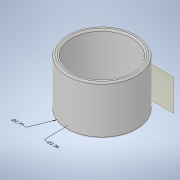
# Autodesk Inventor part: LargeFinderObjectiveCover-V02
Saved by Autodesk Inventor 2021.1 (Build 251245010, 245A)
## iProperties
Created: 2018-09-01
Part Number: LargeFinderObjectiveCover-V02
Material: Generic
Document SubType Name: Modeling
Designer: steele
Density: 1 g/cm^3
Appearance: Default
Author: steele
Autodesk Inventor part; units mm, degrees
ref_plane "YZ Plane" through (0, 0, 0) normal (1, 0, 0) x (0, 1, 0)
ref_plane "XZ Plane" through (0, 0, 0) normal (0, 1, 0) x (-1, 0, 0)
sketch "Sketch1" plane through (0, 0, 0) normal (0, 1, 0) x (-1, 0, 0)
  circle A0 centre (0, 0) radius 35.1155
  dimension "d0" = 70.231
  constraints: 1 centre point, 1 coincident
  measures "d0" diameter of A0
extrude "Extrusion1" add sketch "Sketch1" along normal blind 4.7625
sketch "Sketch2" plane through (0, 4.7625, 0) normal (0, 1, 0) x (1, 0, 0)
  circle A0 centre (0, 0) radius 35.1155
  circle A1 centre (0, 0) radius 30.353
  dimension "d4" = 60.706
  dimension "d5" = 70.231
  constraints: 2 centre point, 1 coincident
  measures "d4" diameter of A1
  measures "d5" diameter of A0
extrude "Extrusion3" add sketch "Sketch2" along normal blind 44.45
ref_plane "Work Plane1" through (0, 0, -35.1155) normal (0, 0, 1) x (1, 0, 0)
sketch "Sketch5" plane through (0, 0, -35.1155) normal (0, 0, 1) x (1, 0, 0)
  line L0 (-35.1155, 0) -> (-35.1155, 49.2125) projected
  line L1 (35.1155, 0) -> (35.1155, 49.2125) projected
  line L2 (35.1155, 24.6063) -> (-35.1155, 24.6063) construction
  line L3 (-14.5772, 19.5263) -> (-16.545, 19.5263)
  line L4 (-16.545, 19.5263) -> (-16.545, 19.0075)
  line L5 (-16.545, 19.0075) -> (-15.8987, 19.0075)
  line L6 (-15.8987, 19.0075) -> (-15.8987, 14.965)
  line L7 (-15.8987, 14.965) -> (-16.545, 14.965)
  line L8 (-16.545, 14.965) -> (-16.545, 14.4462)
  line L9 (-16.545, 14.4462) -> (-14.5772, 14.4462)
  line L10 (-14.5772, 14.4462) -> (-14.5772, 14.965)
  line L11 (-14.5772, 14.965) -> (-15.2235, 14.965)
  line L12 (-15.2235, 14.965) -> (-15.2235, 19.0075)
  line L13 (-15.2235, 19.0075) -> (-14.5772, 19.0075)
  line L14 (-14.5772, 19.0075) -> (-14.5772, 19.5263)
  spline S0 degree 2 poles (-9.736, 16.9904) (-9.736, 17.6861) (-10.3, 18.8058) (-10.7734, 19.1187) knots 0 0 0 1 2 2 2
  spline S1 degree 2 poles (-10.7734, 19.1187) (-11.1604, 19.3616) (-11.9549, 19.5263) (-12.5724, 19.5263) knots 0 0 0 1 2 2 2
  line L15 (-12.5724, 19.5263) -> (-13.7415, 19.5263)
  line L16 (-13.7415, 19.5263) -> (-13.7415, 14.4462)
  line L17 (-13.7415, 14.4462) -> (-12.5847, 14.4462)
  spline S2 degree 2 poles (-12.5847, 14.4462) (-11.8684, 14.4462) (-11.0533, 14.6603) (-10.7652, 14.8497) knots 0 0 0 1 2 2 2
  spline S3 degree 2 poles (-10.7652, 14.8497) (-10.2753, 15.1749) (-9.736, 16.2494) (-9.736, 16.9904) knots 0 0 0 1 2 2 2
  spline S4 degree 2 poles (-10.4399, 16.9821) (-10.4399, 16.3976) (-10.8269, 15.5701) (-11.2098, 15.3355) knots 0 0 0 1 2 2 2
  spline S5 degree 2 poles (-11.2098, 15.3355) (-11.4815, 15.1749) (-12.0948, 15.0308) (-12.5518, 15.0308) knots 0 0 0 1 2 2 2
  line L18 (-12.5518, 15.0308) -> (-13.0664, 15.0308)
  line L19 (-13.0664, 15.0308) -> (-13.0664, 18.9417)
  line L20 (-13.0664, 18.9417) -> (-12.5518, 18.9417)
  spline S6 degree 2 poles (-12.5518, 18.9417) (-12.1031, 18.9417) (-11.4238, 18.7976) (-11.148, 18.6041) knots 0 0 0 1 2 2 2
  spline S7 degree 2 poles (-11.148, 18.6041) (-10.794, 18.3653) (-10.4399, 17.5749) (-10.4399, 16.9821) knots 0 0 0 1 2 2 2
  line L21 (-3.5115, 19.5263) -> (-4.3266, 19.5263)
  line L22 (-4.3266, 19.5263) -> (-4.3266, 18.5547)
  line L23 (-4.3266, 18.5547) -> (-3.5115, 18.5547)
  line L24 (-3.5115, 18.5547) -> (-3.5115, 19.5263)
  line L25 (-3.5115, 16.6857) -> (-4.3266, 16.6857)
  line L26 (-4.3266, 16.6857) -> (-4.3266, 15.7142)
  line L27 (-4.3266, 15.7142) -> (-3.5115, 15.7142)
  line L28 (-3.5115, 15.7142) -> (-3.5115, 16.6857)
  line L29 (3.0011, 19.5263) -> (-0.1317, 19.5263)
  line L30 (-0.1317, 19.5263) -> (-0.1317, 18.8058)
  spline S8 degree 2 poles (-0.1317, 18.8058) (0.2058, 18.4888) (0.8069, 17.9002) (1.095, 17.5832) knots 0 0 0 1 2 2 2
  spline S9 degree 2 poles (1.095, 17.5832) (1.6755, 16.9451) (2.0995, 16.1794) (2.0995, 15.7718) knots 0 0 0 1 2 2 2
  spline S10 degree 2 poles (2.0995, 15.7718) (2.0995, 15.5578) (1.9678, 15.2367) (1.8484, 15.1337) knots 0 0 0 1 2 2 2
  spline S11 degree 2 poles (1.8484, 15.1337) (1.729, 15.0308) (1.4161, 14.9279) (1.2268, 14.9279) knots 0 0 0 1 2 2 2
  spline S12 degree 2 poles (1.2268, 14.9279) (1.0456, 14.9279) (0.6751, 15.0185) (0.5064, 15.0885) knots 0 0 0 1 2 2 2
  spline S13 degree 2 poles (0.5064, 15.0885) (0.3623, 15.1461) (0.0947, 15.3108) (0.0123, 15.3684) knots 0 0 0 1 2 2 2
  line L31 (0.0123, 15.3684) -> (-0.0247, 15.3684)
  line L32 (-0.0247, 15.3684) -> (-0.0247, 14.6439)
  spline S14 degree 2 poles (-0.0247, 14.6439) (0.1853, 14.5409) (0.9386, 14.3392) (1.2762, 14.3392) knots 0 0 0 1 2 2 2
  spline S15 degree 2 poles (1.2762, 14.3392) (1.9884, 14.3392) (2.7911, 15.0926) (2.7911, 15.7348) knots 0 0 0 1 2 2 2
  spline S16 degree 2 poles (2.7911, 15.7348) (2.7911, 16.0353) (2.6512, 16.5375) (2.5276, 16.7516) knots 0 0 0 1 2 2 2
  spline S17 degree 2 poles (2.5276, 16.7516) (2.4041, 16.9739) (2.046, 17.4103) (1.8484, 17.6202) knots 0 0 0 1 2 2 2
  spline S18 degree 2 poles (1.8484, 17.6202) (1.5273, 17.9701) (0.741, 18.7194) (0.5064, 18.9376) knots 0 0 0 1 2 2 2
  line L33 (0.5064, 18.9376) -> (3.0011, 18.9376)
  line L34 (3.0011, 18.9376) -> (3.0011, 19.5263)
  line L35 (4.7712, 19.5263) -> (3.9561, 19.5263)
  line L36 (3.9561, 19.5263) -> (3.9561, 18.5547)
  line L37 (3.9561, 18.5547) -> (4.7712, 18.5547)
  line L38 (4.7712, 18.5547) -> (4.7712, 19.5263)
  spline S19 degree 2 poles (7.1672, 14.9279) (6.9819, 14.9279) (6.6155, 15.0185) (6.4385, 15.0885) knots 0 0 0 1 2 2 2
  spline S20 degree 2 poles (6.4385, 15.0885) (6.2738, 15.1584) (6.031, 15.3066) (5.9363, 15.3725) knots 0 0 0 1 2 2 2
  line L39 (5.9363, 15.3725) -> (5.8951, 15.3725)
  line L40 (5.8951, 15.3725) -> (5.8951, 14.6521)
  spline S21 degree 2 poles (5.8951, 14.6521) (6.1174, 14.5327) (6.879, 14.3392) (7.2207, 14.3392) knots 0 0 0 1 2 2 2
  spline S22 degree 2 poles (7.2207, 14.3392) (7.5665, 14.3392) (8.0811, 14.4792) (8.291, 14.6274) knots 0 0 0 1 2 2 2
  spline S23 degree 2 poles (8.291, 14.6274) (8.5133, 14.7879) (8.7439, 15.2531) (8.7439, 15.566) knots 0 0 0 1 2 2 2
  spline S24 degree 2 poles (8.7439, 15.566) (8.7439, 15.9859) (8.1922, 16.6199) (7.8053, 16.7022) knots 0 0 0 1 2 2 2
  line L41 (7.8053, 16.7022) -> (7.8053, 16.7516)
  spline S25 degree 2 poles (7.8053, 16.7516) (7.9658, 16.7845) (8.3322, 16.9327) (8.4886, 17.0809) knots 0 0 0 1 2 2 2
  spline S26 degree 2 poles (8.4886, 17.0809) (8.6451, 17.225) (8.8427, 17.6861) (8.8427, 18.0195) knots 0 0 0 1 2 2 2
  spline S27 degree 2 poles (8.8427, 18.0195) (8.8427, 18.3612) (8.608, 18.9417) (8.3939, 19.164) knots 0 0 0 1 2 2 2
  spline S28 degree 2 poles (8.3939, 19.164) (8.1716, 19.3945) (7.5418, 19.6333) (7.1425, 19.6333) knots 0 0 0 1 2 2 2
  spline S29 degree 2 poles (7.1425, 19.6333) (6.7596, 19.6333) (6.0104, 19.448) (5.7551, 19.3204) knots 0 0 0 1 2 2 2
  line L42 (5.7551, 19.3204) -> (5.7551, 18.6)
  line L43 (5.7551, 18.6) -> (5.8045, 18.6)
  spline S30 degree 2 poles (5.8045, 18.6) (6.0186, 18.7564) (6.7431, 19.0446) (7.1013, 19.0446) knots 0 0 0 1 2 2 2
  spline S31 degree 2 poles (7.1013, 19.0446) (7.3112, 19.0446) (7.7312, 18.9129) (7.8711, 18.7605) knots 0 0 0 1 2 2 2
  spline S32 degree 2 poles (7.8711, 18.7605) (8.007, 18.6082) (8.1511, 18.246) (8.1511, 17.9701) knots 0 0 0 1 2 2 2
  spline S33 degree 2 poles (8.1511, 17.9701) (8.1511, 17.6943) (7.9905, 17.3362) (7.8464, 17.2333) knots 0 0 0 1 2 2 2
  spline S34 degree 2 poles (7.8464, 17.2333) (7.7023, 17.1303) (7.3112, 17.0521) (7.0807, 17.0521) knots 0 0 0 1 2 2 2
  line L44 (7.0807, 17.0521) -> (6.7925, 17.0521)
  line L45 (6.7925, 17.0521) -> (6.7925, 16.4881)
  line L46 (6.7925, 16.4881) -> (7.019, 16.4881)
  spline S35 degree 2 poles (7.019, 16.4881) (7.4759, 16.4881) (8.0523, 16.0518) (8.0523, 15.636) knots 0 0 0 1 2 2 2
  spline S36 degree 2 poles (8.0523, 15.636) (8.0523, 15.4425) (7.9041, 15.1667) (7.7847, 15.0843) knots 0 0 0 1 2 2 2
  spline S37 degree 2 poles (7.7847, 15.0843) (7.6571, 14.9979) (7.3442, 14.9279) (7.1672, 14.9279) knots 0 0 0 1 2 2 2
  spline S38 degree 2 poles (9.4684, 16.097) (9.4684, 15.706) (9.7236, 15.0555) (9.9459, 14.8209) knots 0 0 0 1 2 2 2
  spline S39 degree 2 poles (9.9459, 14.8209) (10.1559, 14.5945) (10.7693, 14.3433) (11.0821, 14.3433) knots 0 0 0 1 2 2 2
  spline S40 degree 2 poles (11.0821, 14.3433) (11.4321, 14.3433) (12.0002, 14.578) (12.2101, 14.8003) knots 0 0 0 1 2 2 2
  spline S41 degree 2 poles (12.2101, 14.8003) (12.4736, 15.0802) (12.7618, 15.9859) (12.7618, 16.6816) knots 0 0 0 1 2 2 2
  spline S42 degree 2 poles (12.7618, 16.6816) (12.7618, 17.3115) (12.4777, 18.4394) (12.2019, 18.8141) knots 0 0 0 1 2 2 2
  spline S43 degree 2 poles (12.2019, 18.8141) (11.9096, 19.2093) (11.0863, 19.6251) (10.4852, 19.6251) knots 0 0 0 1 2 2 2
  spline S44 degree 2 poles (10.4852, 19.6251) (10.3494, 19.6251) (10.0406, 19.5962) (9.9089, 19.5551) knots 0 0 0 1 2 2 2
  line L47 (9.9089, 19.5551) -> (9.9089, 18.9005)
  line L48 (9.9089, 18.9005) -> (9.9418, 18.9005)
  spline S45 degree 2 poles (9.9418, 18.9005) (10.0283, 18.9499) (10.3905, 19.0364) (10.5758, 19.0364) knots 0 0 0 1 2 2 2
  spline S46 degree 2 poles (10.5758, 19.0364) (11.2427, 19.0364) (12.0043, 18.1554) (12.0578, 17.3403) knots 0 0 0 1 2 2 2
  spline S47 degree 2 poles (12.0578, 17.3403) (11.7861, 17.5255) (11.2921, 17.6943) (10.9998, 17.6943) knots 0 0 0 1 2 2 2
  spline S48 degree 2 poles (10.9998, 17.6943) (10.7199, 17.6943) (10.2547, 17.5708) (10.02, 17.3938) knots 0 0 0 1 2 2 2
  spline S49 degree 2 poles (10.02, 17.3938) (9.7483, 17.1839) (9.4684, 16.5458) (9.4684, 16.097) knots 0 0 0 1 2 2 2
  spline S50 degree 2 poles (12.0743, 16.5293) (12.0743, 16.0147) (11.8849, 15.3643) (11.7161, 15.1873) knots 0 0 0 1 2 2 2
  spline S51 degree 2 poles (11.7161, 15.1873) (11.5679, 15.0226) (11.2592, 14.8991) (11.078, 14.8991) knots 0 0 0 1 2 2 2
  spline S52 degree 2 poles (11.078, 14.8991) (10.6581, 14.8991) (10.16, 15.5001) (10.16, 16.0682) knots 0 0 0 1 2 2 2
  spline S53 degree 2 poles (10.16, 16.0682) (10.16, 16.3893) (10.3247, 16.8051) (10.5058, 16.9533) knots 0 0 0 1 2 2 2
  spline S54 degree 2 poles (10.5058, 16.9533) (10.6375, 17.0604) (10.9628, 17.1303) (11.1521, 17.1303) knots 0 0 0 1 2 2 2
  spline S55 degree 2 poles (11.1521, 17.1303) (11.3703, 17.1303) (11.8725, 16.978) (12.0619, 16.8504) knots 0 0 0 1 2 2 2
  spline S56 degree 2 poles (12.0619, 16.8504) (12.066, 16.801) (12.0743, 16.6322) (12.0743, 16.5293) knots 0 0 0 1 2 2 2
  spline S57 degree 2 poles (16.582, 16.9862) (16.582, 18.353) (15.7875, 19.6333) (14.9601, 19.6333) knots 0 0 0 1 2 2 2
  spline S58 degree 2 poles (14.9601, 19.6333) (14.1203, 19.6333) (13.334, 18.3283) (13.334, 16.9904) knots 0 0 0 1 2 2 2
  spline S59 degree 2 poles (13.334, 16.9904) (13.334, 15.6154) (14.1285, 14.3433) (14.9601, 14.3433) knots 0 0 0 1 2 2 2
  spline S60 degree 2 poles (14.9601, 14.3433) (15.7958, 14.3433) (16.582, 15.6607) (16.582, 16.9862) knots 0 0 0 1 2 2 2
  spline S61 degree 2 poles (15.7093, 18.5341) (15.8081, 18.283) (15.8904, 17.5091) (15.8904, 16.9862) knots 0 0 0 1 2 2 2
  spline S62 degree 2 poles (15.8904, 16.9862) (15.8904, 16.4634) (15.8081, 15.6936) (15.7052, 15.4343) knots 0 0 0 1 2 2 2
  spline S63 degree 2 poles (15.7052, 15.4343) (15.6023, 15.1749) (15.2441, 14.9073) (14.9601, 14.9073) knots 0 0 0 1 2 2 2
  spline S64 degree 2 poles (14.9601, 14.9073) (14.676, 14.9073) (14.3096, 15.1749) (14.2026, 15.4425) knots 0 0 0 1 2 2 2
  spline S65 degree 2 poles (14.2026, 15.4425) (14.0997, 15.7018) (14.0256, 16.4922) (14.0256, 16.9904) knots 0 0 0 1 2 2 2
  spline S66 degree 2 poles (14.0256, 16.9904) (14.0256, 17.5255) (14.0914, 18.2418) (14.1985, 18.5218) knots 0 0 0 1 2 2 2
  spline S67 degree 2 poles (14.1985, 18.5218) (14.2973, 18.7852) (14.6637, 19.0693) (14.9601, 19.0693) knots 0 0 0 1 2 2 2
  spline S68 degree 2 poles (14.9601, 19.0693) (15.24, 19.0693) (15.6064, 18.8017) (15.7093, 18.5341) knots 0 0 0 1 2 2 2
  spline S69 degree 2 poles (-12.8317, 23.4156) (-12.5436, 23.7532) (-12.2225, 24.7412) (-12.2225, 25.3752) knots 0 0 0 1 2 2 2
  spline S70 degree 2 poles (-12.2225, 25.3752) (-12.2225, 25.9927) (-12.5353, 26.993) (-12.8317, 27.3306) knots 0 0 0 1 2 2 2
  spline S71 degree 2 poles (-12.8317, 27.3306) (-13.1446, 27.6846) (-13.9721, 28.0222) (-14.4702, 28.0222) knots 0 0 0 1 2 2 2
  spline S72 degree 2 poles (-14.4702, 28.0222) (-14.9848, 28.0222) (-15.8081, 27.6723) (-16.1086, 27.3306) knots 0 0 0 1 2 2 2
  spline S73 degree 2 poles (-16.1086, 27.3306) (-16.4009, 26.993) (-16.7138, 26.0009) (-16.7138, 25.3752) knots 0 0 0 1 2 2 2
  spline S74 degree 2 poles (-16.7138, 25.3752) (-16.7138, 24.7371) (-16.3968, 23.7655) (-16.1045, 23.4156) knots 0 0 0 1 2 2 2
  spline S75 degree 2 poles (-16.1045, 23.4156) (-15.8081, 23.078) (-14.9806, 22.7281) (-14.4702, 22.7281) knots 0 0 0 1 2 2 2
  spline S76 degree 2 poles (-14.4702, 22.7281) (-13.9515, 22.7281) (-13.1199, 23.0904) (-12.8317, 23.4156) knots 0 0 0 1 2 2 2
  spline S77 degree 2 poles (-12.9264, 25.3752) (-12.9264, 24.8729) (-13.1446, 24.0949) (-13.3422, 23.8396) knots 0 0 0 1 2 2 2
  spline S78 degree 2 poles (-13.3422, 23.8396) (-13.5439, 23.5762) (-14.112, 23.3127) (-14.4661, 23.3127) knots 0 0 0 1 2 2 2
  spline S79 degree 2 poles (-14.4661, 23.3127) (-14.8324, 23.3127) (-15.3841, 23.5679) (-15.594, 23.8396) knots 0 0 0 1 2 2 2
  spline S80 degree 2 poles (-15.594, 23.8396) (-15.7958, 24.099) (-16.0098, 24.8812) (-16.0098, 25.3752) knots 0 0 0 1 2 2 2
  spline S81 degree 2 poles (-16.0098, 25.3752) (-16.0098, 26.3755) (-15.17, 27.4376) (-14.4661, 27.4376) knots 0 0 0 1 2 2 2
  spline S82 degree 2 poles (-14.4661, 27.4376) (-13.7621, 27.4376) (-12.9264, 26.3755) (-12.9264, 25.3752) knots 0 0 0 1 2 2 2
  spline S83 degree 2 poles (-7.4759, 25.3793) (-7.4759, 26.075) (-8.0399, 27.1947) (-8.5133, 27.5076) knots 0 0 0 1 2 2 2
  spline S84 degree 2 poles (-8.5133, 27.5076) (-8.9003, 27.7505) (-9.6948, 27.9152) (-10.3123, 27.9152) knots 0 0 0 1 2 2 2
  line L49 (-10.3123, 27.9152) -> (-11.4815, 27.9152)
  line L50 (-11.4815, 27.9152) -> (-11.4815, 22.8352)
  line L51 (-11.4815, 22.8352) -> (-10.3247, 22.8352)
  spline S85 degree 2 poles (-10.3247, 22.8352) (-9.6084, 22.8352) (-8.7933, 23.0492) (-8.5051, 23.2386) knots 0 0 0 1 2 2 2
  spline S86 degree 2 poles (-8.5051, 23.2386) (-8.0152, 23.5638) (-7.4759, 24.6383) (-7.4759, 25.3793) knots 0 0 0 1 2 2 2
  spline S87 degree 2 poles (-8.1799, 25.371) (-8.1799, 24.7865) (-8.5668, 23.959) (-8.9497, 23.7244) knots 0 0 0 1 2 2 2
  spline S88 degree 2 poles (-8.9497, 23.7244) (-9.2214, 23.5638) (-9.8348, 23.4197) (-10.2917, 23.4197) knots 0 0 0 1 2 2 2
  line L52 (-10.2917, 23.4197) -> (-10.8063, 23.4197)
  line L53 (-10.8063, 23.4197) -> (-10.8063, 27.3306)
  line L54 (-10.8063, 27.3306) -> (-10.2917, 27.3306)
  spline S89 degree 2 poles (-10.2917, 27.3306) (-9.843, 27.3306) (-9.1638, 27.1865) (-8.8879, 26.993) knots 0 0 0 1 2 2 2
  spline S90 degree 2 poles (-8.8879, 26.993) (-8.5339, 26.7542) (-8.1799, 25.9638) (-8.1799, 25.371) knots 0 0 0 1 2 2 2
  line L55 (-3.4333, 27.9152) -> (-4.2484, 27.9152)
  line L56 (-4.2484, 27.9152) -> (-4.2484, 26.9436)
  line L57 (-4.2484, 26.9436) -> (-3.4333, 26.9436)
  line L58 (-3.4333, 26.9436) -> (-3.4333, 27.9152)
  line L59 (-3.4333, 25.0746) -> (-4.2484, 25.0746)
  line L60 (-4.2484, 25.0746) -> (-4.2484, 24.1031)
  line L61 (-4.2484, 24.1031) -> (-3.4333, 24.1031)
  line L62 (-3.4333, 24.1031) -> (-3.4333, 25.0746)
  line L63 (3.0793, 27.9152) -> (-0.0535, 27.9152)
  line L64 (-0.0535, 27.9152) -> (-0.0535, 27.1947)
  spline S91 degree 2 poles (-0.0535, 27.1947) (0.2841, 26.8777) (0.8851, 26.2891) (1.1733, 25.9721) knots 0 0 0 1 2 2 2
  spline S92 degree 2 poles (1.1733, 25.9721) (1.7537, 25.334) (2.1777, 24.5683) (2.1777, 24.1607) knots 0 0 0 1 2 2 2
  spline S93 degree 2 poles (2.1777, 24.1607) (2.1777, 23.9467) (2.046, 23.6256) (1.9266, 23.5226) knots 0 0 0 1 2 2 2
  spline S94 degree 2 poles (1.9266, 23.5226) (1.8072, 23.4197) (1.4944, 23.3168) (1.305, 23.3168) knots 0 0 0 1 2 2 2
  spline S95 degree 2 poles (1.305, 23.3168) (1.1239, 23.3168) (0.7534, 23.4074) (0.5846, 23.4774) knots 0 0 0 1 2 2 2
  spline S96 degree 2 poles (0.5846, 23.4774) (0.4405, 23.535) (0.1729, 23.6997) (0.0906, 23.7573) knots 0 0 0 1 2 2 2
  line L65 (0.0906, 23.7573) -> (0.0535, 23.7573)
  line L66 (0.0535, 23.7573) -> (0.0535, 23.0328)
  spline S97 degree 2 poles (0.0535, 23.0328) (0.2635, 22.9298) (1.0168, 22.7281) (1.3544, 22.7281) knots 0 0 0 1 2 2 2
  spline S98 degree 2 poles (1.3544, 22.7281) (2.0666, 22.7281) (2.8693, 23.4815) (2.8693, 24.1237) knots 0 0 0 1 2 2 2
  spline S99 degree 2 poles (2.8693, 24.1237) (2.8693, 24.4242) (2.7294, 24.9264) (2.6059, 25.1405) knots 0 0 0 1 2 2 2
  spline S100 degree 2 poles (2.6059, 25.1405) (2.4824, 25.3628) (2.1242, 25.7992) (1.9266, 26.0091) knots 0 0 0 1 2 2 2
  spline S101 degree 2 poles (1.9266, 26.0091) (1.6055, 26.359) (0.8192, 27.1083) (0.5846, 27.3265) knots 0 0 0 1 2 2 2
  line L67 (0.5846, 27.3265) -> (3.0793, 27.3265)
  line L68 (3.0793, 27.3265) -> (3.0793, 27.9152)
  line L69 (4.8495, 27.9152) -> (4.0344, 27.9152)
  line L70 (4.0344, 27.9152) -> (4.0344, 26.9436)
  line L71 (4.0344, 26.9436) -> (4.8495, 26.9436)
  line L72 (4.8495, 26.9436) -> (4.8495, 27.9152)
  line L73 (9.065, 23.5967) -> (6.8666, 27.9152)
  line L74 (6.8666, 27.9152) -> (6.1421, 27.9152)
  line L75 (6.1421, 27.9152) -> (8.4639, 23.4321)
  line L76 (8.4639, 23.4321) -> (5.8416, 23.4321)
  line L77 (5.8416, 23.4321) -> (5.8416, 22.8352)
  line L78 (5.8416, 22.8352) -> (9.065, 22.8352)
  line L79 (9.065, 22.8352) -> (9.065, 23.5967)
  line L80 (12.877, 23.5967) -> (10.6787, 27.9152)
  line L81 (10.6787, 27.9152) -> (9.9542, 27.9152)
  line L82 (9.9542, 27.9152) -> (12.276, 23.4321)
  line L83 (12.276, 23.4321) -> (9.6536, 23.4321)
  line L84 (9.6536, 23.4321) -> (9.6536, 22.8352)
  line L85 (9.6536, 22.8352) -> (12.877, 22.8352)
  line L86 (12.877, 22.8352) -> (12.877, 23.5967)
  spline S102 degree 2 poles (16.6603, 25.3752) (16.6603, 26.7419) (15.8657, 28.0222) (15.0383, 28.0222) knots 0 0 0 1 2 2 2
  spline S103 degree 2 poles (15.0383, 28.0222) (14.1985, 28.0222) (13.4122, 26.7172) (13.4122, 25.3793) knots 0 0 0 1 2 2 2
  spline S104 degree 2 poles (13.4122, 25.3793) (13.4122, 24.0043) (14.2067, 22.7322) (15.0383, 22.7322) knots 0 0 0 1 2 2 2
  spline S105 degree 2 poles (15.0383, 22.7322) (15.874, 22.7322) (16.6603, 24.0496) (16.6603, 25.3752) knots 0 0 0 1 2 2 2
  spline S106 degree 2 poles (15.7875, 26.923) (15.8863, 26.6719) (15.9687, 25.898) (15.9687, 25.3752) knots 0 0 0 1 2 2 2
  spline S107 degree 2 poles (15.9687, 25.3752) (15.9687, 24.8523) (15.8863, 24.0825) (15.7834, 23.8232) knots 0 0 0 1 2 2 2
  spline S108 degree 2 poles (15.7834, 23.8232) (15.6805, 23.5638) (15.3223, 23.2962) (15.0383, 23.2962) knots 0 0 0 1 2 2 2
  spline S109 degree 2 poles (15.0383, 23.2962) (14.7542, 23.2962) (14.3878, 23.5638) (14.2808, 23.8314) knots 0 0 0 1 2 2 2
  spline S110 degree 2 poles (14.2808, 23.8314) (14.1779, 24.0907) (14.1038, 24.8812) (14.1038, 25.3793) knots 0 0 0 1 2 2 2
  spline S111 degree 2 poles (14.1038, 25.3793) (14.1038, 25.9144) (14.1697, 26.6307) (14.2767, 26.9107) knots 0 0 0 1 2 2 2
  spline S112 degree 2 poles (14.2767, 26.9107) (14.3755, 27.1742) (14.7419, 27.4582) (15.0383, 27.4582) knots 0 0 0 1 2 2 2
  spline S113 degree 2 poles (15.0383, 27.4582) (15.3182, 27.4582) (15.6846, 27.1906) (15.7875, 26.923) knots 0 0 0 1 2 2 2
  line L87 (-2.9661, 31.2241) -> (-4.7157, 36.3041)
  line L88 (-4.7157, 36.3041) -> (-5.4443, 36.3041)
  line L89 (-5.4443, 36.3041) -> (-7.1939, 31.2241)
  line L90 (-7.1939, 31.2241) -> (-6.4694, 31.2241)
  line L91 (-6.4694, 31.2241) -> (-5.0615, 35.4437)
  line L92 (-5.0615, 35.4437) -> (-3.6536, 31.2241)
  line L93 (-3.6536, 31.2241) -> (-2.9661, 31.2241)
  line L94 (-0.706, 34.3898) -> (-2.6285, 34.3898)
  line L95 (-2.6285, 34.3898) -> (-2.6285, 33.7723)
  line L96 (-2.6285, 33.7723) -> (-0.706, 33.7723)
  line L97 (-0.706, 33.7723) -> (-0.706, 34.3898)
  spline S114 degree 2 poles (3.1307, 33.7641) (3.1307, 35.1308) (2.3362, 36.4111) (1.5088, 36.4111) knots 0 0 0 1 2 2 2
  spline S115 degree 2 poles (1.5088, 36.4111) (0.669, 36.4111) (-0.1173, 35.1061) (-0.1173, 33.7682) knots 0 0 0 1 2 2 2
  spline S116 degree 2 poles (-0.1173, 33.7682) (-0.1173, 32.3932) (0.6772, 31.1211) (1.5088, 31.1211) knots 0 0 0 1 2 2 2
  spline S117 degree 2 poles (1.5088, 31.1211) (2.3445, 31.1211) (3.1307, 32.4385) (3.1307, 33.7641) knots 0 0 0 1 2 2 2
  spline S118 degree 2 poles (2.258, 35.3119) (2.3568, 35.0608) (2.4391, 34.2869) (2.4391, 33.7641) knots 0 0 0 1 2 2 2
  spline S119 degree 2 poles (2.4391, 33.7641) (2.4391, 33.2412) (2.3568, 32.4714) (2.2539, 32.2121) knots 0 0 0 1 2 2 2
  spline S120 degree 2 poles (2.2539, 32.2121) (2.151, 31.9527) (1.7928, 31.6851) (1.5088, 31.6851) knots 0 0 0 1 2 2 2
  spline S121 degree 2 poles (1.5088, 31.6851) (1.2247, 31.6851) (0.8583, 31.9527) (0.7513, 32.2203) knots 0 0 0 1 2 2 2
  spline S122 degree 2 poles (0.7513, 32.2203) (0.6484, 32.4797) (0.5743, 33.2701) (0.5743, 33.7682) knots 0 0 0 1 2 2 2
  spline S123 degree 2 poles (0.5743, 33.7682) (0.5743, 34.3033) (0.6401, 35.0197) (0.7472, 35.2996) knots 0 0 0 1 2 2 2
  spline S124 degree 2 poles (0.7472, 35.2996) (0.846, 35.5631) (1.2124, 35.8471) (1.5088, 35.8471) knots 0 0 0 1 2 2 2
  spline S125 degree 2 poles (1.5088, 35.8471) (1.7887, 35.8471) (2.1551, 35.5795) (2.258, 35.3119) knots 0 0 0 1 2 2 2
  line L98 (6.914, 36.3041) -> (3.7812, 36.3041)
  line L99 (3.7812, 36.3041) -> (3.7812, 35.5836)
  spline S126 degree 2 poles (3.7812, 35.5836) (4.1188, 35.2667) (4.7198, 34.678) (5.008, 34.361) knots 0 0 0 1 2 2 2
  spline S127 degree 2 poles (5.008, 34.361) (5.5884, 33.7229) (6.0124, 32.9572) (6.0124, 32.5496) knots 0 0 0 1 2 2 2
  spline S128 degree 2 poles (6.0124, 32.5496) (6.0124, 32.3356) (5.8807, 32.0145) (5.7613, 31.9115) knots 0 0 0 1 2 2 2
  spline S129 degree 2 poles (5.7613, 31.9115) (5.6419, 31.8086) (5.3291, 31.7057) (5.1397, 31.7057) knots 0 0 0 1 2 2 2
  spline S130 degree 2 poles (5.1397, 31.7057) (4.9586, 31.7057) (4.5881, 31.7963) (4.4193, 31.8663) knots 0 0 0 1 2 2 2
  spline S131 degree 2 poles (4.4193, 31.8663) (4.2752, 31.9239) (4.0076, 32.0886) (3.9253, 32.1462) knots 0 0 0 1 2 2 2
  line L100 (3.9253, 32.1462) -> (3.8882, 32.1462)
  line L101 (3.8882, 32.1462) -> (3.8882, 31.4217)
  spline S132 degree 2 poles (3.8882, 31.4217) (4.0982, 31.3187) (4.8515, 31.117) (5.1891, 31.117) knots 0 0 0 1 2 2 2
  spline S133 degree 2 poles (5.1891, 31.117) (5.9013, 31.117) (6.704, 31.8704) (6.704, 32.5126) knots 0 0 0 1 2 2 2
  spline S134 degree 2 poles (6.704, 32.5126) (6.704, 32.8131) (6.5641, 33.3153) (6.4406, 33.5294) knots 0 0 0 1 2 2 2
  spline S135 degree 2 poles (6.4406, 33.5294) (6.3171, 33.7517) (5.9589, 34.1881) (5.7613, 34.398) knots 0 0 0 1 2 2 2
  spline S136 degree 2 poles (5.7613, 34.398) (5.4402, 34.7479) (4.6539, 35.4972) (4.4193, 35.7154) knots 0 0 0 1 2 2 2
  line L102 (4.4193, 35.7154) -> (6.914, 35.7154)
  line L103 (6.914, 35.7154) -> (6.914, 36.3041)
  point P0 (0, 0)
  constraints: 2 end point, 2 midpoint, 1 horizontal
emboss "Emboss1" sketch "Sketch5" operation cut depth 1.27 direction (0, 0, -1) wrap yes faces at (-29.3386, 16.4042, -19.2963)
fillet "Fillet1" radius 1.5875 2 edges at (-35.1155, 49.2125, 0) (-30.353, 49.2125, 0)
fillet "Fillet2" radius 1.5875 1 edges at (35.1155, 0, 0)
equation "\"d0\" = lensCoverOD"
equation "\"d2\" = wallThickness"
equation "\"d4\" = lensCoverID"
equation "\"d5\" = lensCoverOD"
equation "\"d9\" = lensCoverLength"
equation "\"d11\" = textDepth"
equation "\"d13\" = filetRadius"
equation "\"d14\" = filetRadius"
equation "\"objectiveOD\" = 60.325"
equation "\"lensCoverLength\" = 44.45"
equation "\"wallThickness\" = 4.7625"
equation "\"lensCoverOD\" = lensCoverID + 2 * wallThickness"
equation "\"clearance\" = 0.381"
equation "\"lensCoverID\" = objectiveOD + clearance"
equation "\"textDepth\" = 1.27"
equation "\"filetRadius\" = 1.5875"
body "Solid1"
